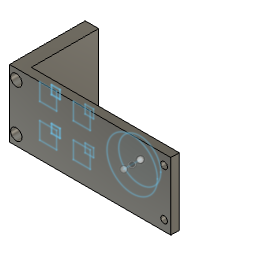
cementform_circle_80x40_plateB (Autodesk Fusion 360 design; units mm, degrees)
Autodesk Fusion 360 part; units mm, degrees
sketch "baseplate" plane through (0, 0, 0) normal (0, 1, 0) x (1, 0, 0)
  line L0 (0, 0) -> (80, 0)
  line L1 (80, 0) -> (80, -40)
  line L2 (80, -40) -> (0, -40)
  line L3 (0, -40) -> (0, 0)
  dimension "d1" = 80
  dimension "d2" = 40
  constraint horizontal L0
  constraint vertical L1
  constraint horizontal L2
  constraint vertical L3
  constraint coincident L0.start L3.end
  measures "d1" distance of L0.start L0.end
  measures "d2" distance of L0.start L2.end
sketch "pryamid_base" plane through (0, 0, 0) normal (0, 1, 0) x (1, 0, 0)
  line L0 (5, -35) -> (15, -35)
  line L1 (15, -35) -> (15, -25)
  line L2 (15, -25) -> (5, -25)
  line L3 (5, -25) -> (5, -35)
  line L4 (35, -35) -> (35, -25)
  line L5 (35, -25) -> (25, -25)
  line L6 (25, -35) -> (35, -35)
  line L7 (25, -25) -> (25, -35)
  line L8 (35, -5) -> (25, -5)
  line L9 (35, -15) -> (35, -5)
  line L10 (15, -5) -> (5, -5)
  line L11 (25, -5) -> (25, -15)
  line L12 (5, -5) -> (5, -15)
  line L13 (5, -15) -> (15, -15)
  line L14 (15, -15) -> (15, -5)
  line L15 (25, -15) -> (35, -15)
  line L16 (55, -15) -> (65, -25)
  circle A0 centre (60, -20) radius 15
  dimension "d3" = 10
  dimension "d4" = 10
  dimension "d5" = 10
  dimension "d6" = 10
  dimension "d11" = 10
  dimension "d12" = 10
  dimension "d13" = 10
  dimension "d14" = 10
  dimension "d48" = 30
  constraint horizontal L0
  constraint vertical L1
  constraint horizontal L2
  constraint vertical L3
  constraint horizontal L6
  constraint vertical L4
  constraint horizontal L5
  constraint vertical L7
  constraint horizontal L13
  constraint vertical L14
  constraint horizontal L10
  constraint vertical L12
  constraint horizontal L15
  constraint vertical L9
  constraint horizontal L8
  constraint vertical L11
  constraint midpoint L16 A0.centre
  measures "d3" distance of L0.start L0.end
  measures "d4" distance of L0.start L2.end
  measures "d5" distance of L6.start L4.start
  measures "d6" distance of L6.start L5.end
  measures "d11" distance of L12.end L13.end
  measures "d12" distance of L12.end L10.end
  measures "d13" distance of L9.start L11.end
  measures "d14" distance of L8.end L11.end
  measures "d48" diameter of A0
ref_plane "WorkPlane1" through (0, 4.5, 0) normal (0, 1, 0) x (0, 0, 1)
sketch "pryamid_offsetplane" plane through (0, 4.5, 0) normal (0, 1, 0) x (1, 0, 0)
  line L0 (7.5, -32.5) -> (12.5, -32.5)
  line L1 (12.5, -32.5) -> (12.5, -27.5)
  line L2 (12.5, -27.5) -> (7.5, -27.5)
  line L3 (7.5, -27.5) -> (7.5, -32.5)
  line L4 (27.5, -27.5) -> (27.5, -32.5)
  line L5 (32.5, -32.5) -> (32.5, -27.5)
  line L6 (27.5, -32.5) -> (32.5, -32.5)
  line L7 (32.5, -27.5) -> (27.5, -27.5)
  line L8 (7.5, -27.5) -> (7.5, -32.5)
  line L9 (12.5, -32.5) -> (12.5, -27.5)
  line L10 (7.5, -32.5) -> (12.5, -32.5)
  line L11 (12.5, -27.5) -> (7.5, -27.5)
  line L12 (27.5, -7.5) -> (27.5, -12.5)
  line L13 (12.5, -12.5) -> (12.5, -7.5)
  line L14 (12.5, -7.5) -> (7.5, -7.5)
  line L15 (7.5, -7.5) -> (7.5, -12.5)
  line L16 (7.5, -12.5) -> (12.5, -12.5)
  line L17 (32.5, -7.5) -> (27.5, -7.5)
  line L18 (27.5, -12.5) -> (32.5, -12.5)
  line L19 (12.5, -7.5) -> (7.5, -7.5)
  line L20 (32.5, -12.5) -> (32.5, -7.5)
  line L21 (12.5, -12.5) -> (12.5, -7.5)
  line L22 (7.5, -12.5) -> (12.5, -12.5)
  line L23 (7.5, -7.5) -> (7.5, -12.5)
  circle A0 centre (60, -20) radius 12.5
  dimension "d49" = 25
  constraint vertical L1
  constraint horizontal L2
  constraint vertical L5
  constraint horizontal L7
  constraint vertical L9
  constraint horizontal L11
  constraint vertical L21
  constraint horizontal L19
  constraint vertical L20
  constraint horizontal L17
  constraint vertical L13
  constraint horizontal L14
  measures "d49" diameter of A0
extrude "Extrude1" add sketch "baseplate" against normal blind 5
loft "Loft1" add profiles "pryamid_base", "pryamid_offsetplane" section 1 contours L0 L1 L2 L3 section 2 contours L0 L1 L2 L3 L8 L9 L10 L11
loft "Loft2" add profiles "pryamid_base", "pryamid_offsetplane" section 1 contours L4 L5 L6 L7 section 2 contours L4 L5 L6 L7
sketch "sidewall" plane through (0, 0, 0) normal (0, 1, 0) x (1, 0, 0)
  line L0 (0, 0) -> (-8, 0)
  line L1 (-8, 0) -> (-8, -40)
  line L2 (-8, -40) -> (0, -40)
  line L3 (0, -40) -> (0, 0)
  dimension "d22" = 8
  constraint horizontal L0
  constraint vertical L1
  constraint horizontal L2
  constraint vertical L3
  constraint coincident L0.start L3.end
  measures "d22" distance of L1.end L2.end
extrude "Extrude2" add sketch "sidewall" along normal blind 40 and the other way blind 5
sketch "sidemount" plane through (0, 0, 0) normal (0, 1, 0) x (1, 0, 0)
  line L0 (80, 0) -> (88, 0)
  line L1 (88, 0) -> (88, -40)
  line L2 (88, -40) -> (80, -40)
  line L3 (80, -40) -> (80, 0)
  constraint horizontal L0
  constraint vertical L1
  constraint horizontal L2
  constraint vertical L3
extrude "Extrude3" add sketch "sidemount" against normal blind 5
sketch "holes" plane through (0, -5, 0) normal (0, -1, 0) x (1, 0, 0)
  line L0 (88, 40) -> (-8, 40)
  line L1 (-8, 40) -> (-8, 0)
  line L2 (-8, 0) -> (88, 0)
  line L3 (88, 0) -> (88, 40)
  line L4 (-8, 0) -> (-4, 0)
  line L5 (-8, 6) -> (-8, 0)
  line L6 (-4, 40) -> (-8, 40)
  line L7 (-8, 40) -> (-8, 34)
  circle A0 centre (-4, 34) radius 2
  circle A1 centre (-4, 6) radius 2
  circle A2 centre (-4, 34) radius 3.4
  circle A3 centre (-4, 6) radius 3.4
  dimension "d29" = 6
  dimension "d30" = 4
  dimension "d31" = 4
  dimension "d32" = 6.8
  dimension "d33" = 6.8
  constraint horizontal L4
  constraint vertical L5
  constraint coincident L1.end L2.start
  constraint horizontal L6
  constraint vertical L7
  constraint coincident L0 L6.start
  constraint concentric A0 A2
  constraint concentric A1 A3
  measures "d29" distance of L6.start A0.centre
  measures "d30" diameter of A0
  measures "d31" diameter of A1
  measures "d32" diameter of A2
  measures "d33" diameter of A3
extrude "Extrude4" cut sketch "holes" against normal blind 51 contours A0 | A1
extrude "Extrude5" cut sketch "holes" against normal blind 5 contours A2 | A3
sketch "holes (1)" plane through (0, -5, 0) normal (0, -1, 0) x (1, 0, 0)
  circle A0 centre (84, 34) radius 2
  circle A1 centre (84, 6) radius 2
  circle A2 centre (84, 34) radius 3.4
  circle A3 centre (84, 6) radius 3.4
  dimension "d42" = 4
  dimension "d43" = 4
  dimension "d44" = 6.8
  dimension "d45" = 6.8
  constraint concentric A0 A2
  constraint concentric A1 A3
  measures "d42" diameter of A0
  measures "d43" diameter of A1
  measures "d44" diameter of A2
  measures "d45" diameter of A3
extrude "Extrude6" cut sketch "holes (1)" against normal blind 16 contours A0 | A1
loft "Loft9" add profiles "pryamid_offsetplane", "pryamid_base" section 1 contours L13 L14 L15 L16 L19 L21 L22 L23 section 2 contours L10 L12 L13 L14
loft "Loft10" add profiles "pryamid_base", "pryamid_offsetplane" section 1 contours L8 L9 L11 L15 section 2 contours L12 L17 L18 L20
loft "Loft11" add profiles "pryamid_offsetplane", "pryamid_base" section 1 contours A0 section 2 contours A0
